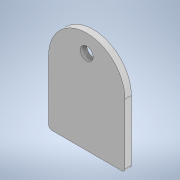
# Autodesk Inventor part: 2 Stage Climer in a box lower bracket
Saved by Autodesk Inventor 2022 (Build 260153000, 153)
## iProperties
Created: 2022-02-15
Part Number: 2 Stage Climer in a box lower bracket
Material: Generic
Document SubType Name: Modeling
Designer: hawle
Density: 1 g/cm^3
Appearance: Default
Author: hawle
Autodesk Inventor part; units mm, degrees
ref_plane "YZ Plane" through (0, 0, 0) normal (1, 0, 0) x (0, 1, 0)
ref_plane "XZ Plane" through (0, 0, 0) normal (0, 1, 0) x (-1, 0, 0)
ref_plane "XY Plane" through (0, 0, 0) normal (0, 0, 1) x (1, 0, 0)
sketch "Sketch1" plane through (0, 0, 0) normal (0, 0, 1) x (1, 0, 0)
  circle A0 centre (-9.1291, -65.9913) radius 6.35
  line L0 (3.5709, -48.3129) -> (3.5709, -48.3129)
  line L1 (28.9709, -86.4129) -> (28.9709, -146.7379)
  line L2 (25.7959, -149.9129) -> (-44.0541, -149.9129)
  line L3 (-47.2291, -146.7379) -> (-47.2291, -86.4129)
  arc A1 (25.7959, -149.9129) -> (28.9709, -146.7379) centre (25.7959, -146.7379) ccw
  arc A2 (-47.2291, -146.7379) -> (-44.0541, -149.9129) centre (-44.0541, -146.7379) ccw
  line L4 (-9.1291, -48.3129) -> (-9.1291, -48.3129)
  arc A3 (-9.1291, -48.3129) -> (-47.2291, -86.4129) centre (-9.1291, -86.4129) ccw
  arc A4 (28.9709, -86.4129) -> (-9.1291, -48.3129) centre (-9.1291, -86.4129) ccw
  point P0 (0, 0)
  point P1 (28.9709, -149.9129)
  point P2 (-47.2291, -149.9129)
  point P3 (28.9709, -73.7129)
  dimension "d0" = 12.7
  dimension "d1" = 76.2
  dimension "d3" = 83.9216
  dimension "d4" = 38.1
  dimension "d11" = 101.6
  dimension "d12" = 38.1
  constraints: 10 end point, 8 point on circle, 8 tangent, 5 centre point, 5 point on line, 2 horizontal, 2 parallel, 1 concentric, 1 perpendicular
  measures "d0" diameter of A0
  measures "d1" distance of point (28.971, -149.913) point (-47.229, -149.913)
  measures "d3" distance from line of L2 A0.centre
  measures "d4" distance from line of L3 A0.centre
  measures "d11" distance between parallel lines of L2 L4
  measures "d12" radius of A3
extrude "Extrusion1" add sketch "Sketch1" along normal blind 6.35
body "Solid1"
